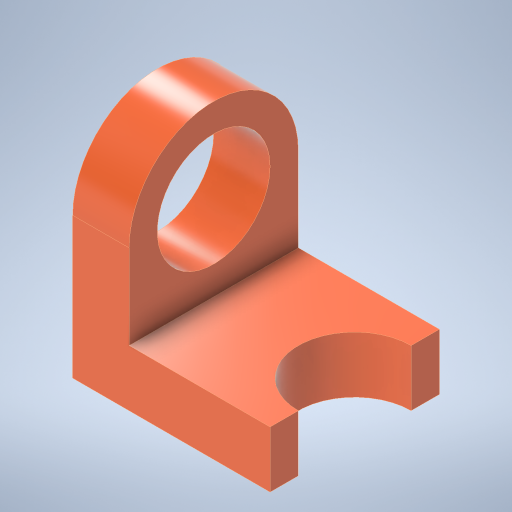
# Autodesk Inventor part: atividade
Saved by Autodesk Inventor 2024 (Build 280153000, 153)
## iProperties
Created: 2023-09-18
Part Number: atividade
Material: Generic
Document SubType Name: Modeling
Designer: LORAC
Density: 1 g/cm^3
Appearance: Smooth - Light Orange
Author: LORAC
Autodesk Inventor part; units mm, degrees
ref_plane "YZ Plane" through (0, 0, 0) normal (1, 0, 0) x (0, 1, 0)
ref_plane "XZ Plane" through (0, 0, 0) normal (0, 1, 0) x (-1, 0, 0)
ref_plane "XY Plane" through (0, 0, 0) normal (0, 0, 1) x (1, 0, 0)
sketch "Sketch1" plane through (0, 0, 0) normal (0, 1, 0) x (-1, 0, 0)
  line L0 (15, 17.5) -> (-15, 17.5)
  line L1 (-15, 17.5) -> (-15, -17.5)
  line L2 (-15, -17.5) -> (15, -17.5)
  line L3 (15, -17.5) -> (15, 17.5)
  line L4 (15, 17.5) -> (-15, -17.5) construction
  line L5 (-15, 17.5) -> (15, -17.5) construction
  arc A0 (-10, 17.5) -> (10, 17.5) centre (0, 17.5) ccw
  point P0 (0, 0)
  dimension "d0" = 30
  dimension "d1" = 35
  dimension "d2" = 20
  constraints: 12 end point, 3 midpoint, 2 parallel, 2 point on circle, 2 point on line, 1 centre point, 1 horizontal, 1 perpendicular
  measures "d0" distance of L2.end L1.end
  measures "d1" distance of L1.end L0.end
  measures "d2" diameter of A0
extrude "Extrusion1" add sketch "Sketch1" along normal blind 10 contours L3 L2 L1 L0 A0
sketch "Sketch2" plane through (0, 10, 0) normal (0, 1, 0) x (1, 0, 0)
  line L0 (15, 17.5) -> (-15, 17.5) projected
  line L1 (15, 17.5) -> (-15, 17.5)
  line L2 (-15, 17.5) -> (-15, 7.5)
  line L3 (-15, 7.5) -> (15, 7.5)
  line L4 (15, 7.5) -> (15, 17.5)
  point P0 (0, 0)
  dimension "d5" = 30
  dimension "d6" = 10
  constraints: 8 end point, 2 parallel, 1 horizontal, 1 perpendicular
  measures "d5" distance of L3.end L2.end
  measures "d6" distance of L2.end L1.end
extrude "Extrusion2" add sketch "Sketch2" along normal blind 15
sketch "Sketch3" plane through (-15, 10, -7.5) normal (0, 0, 1) x (1, 0, 0)
  line L0 (0, 15) -> (30, 15) projected
  arc A0 (30, 15) -> (0, 15) centre (15, 15) ccw
  point P0 (15, -10)
  constraints: 2 end point, 2 point on circle, 1 centre point, 1 midpoint
extrude "Extrusion3" add sketch "Sketch3" against normal blind 10
sketch "Sketch4" plane through (-15, 10, -7.5) normal (0, 0, 1) x (1, 0, 0)
  arc A0 (30, 15) -> (0, 15) centre (15, 15) ccw projected
  circle A1 centre (15, 15) radius 10
  point P0 (15, -10)
  dimension "d12" = 20
  constraints: 1 centre point, 1 coincident
  measures "d12" diameter of A1
extrude "Extrusion4" cut sketch "Sketch4" against normal blind 10
body "Solid1"
